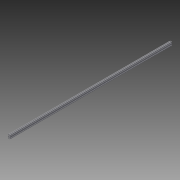
# Autodesk Inventor part: hfs5-2040
Saved by Autodesk Inventor 2013 (Build 170138000, 138)
## iProperties
Created: 2013-06-19
Part Number: hfs5-2040
Material: Generic
Document SubType Name: Modeling
Designer: Brett
Density: 1 g/cm^3
Author: Brett
Autodesk Inventor part; units mm, degrees
ref_plane "YZ Plane" through (0, 0, 0) normal (1, 0, 0) x (0, 1, 0)
ref_plane "XZ Plane" through (0, 0, 0) normal (0, 1, 0) x (-1, 0, 0)
ref_plane "XY Plane" through (0, 0, 0) normal (0, 0, 1) x (1, 0, 0)
sketch "Sketch1" plane through (0, 0, 0) normal (0, 0, 1) x (1, 0, 0)
  circle A0 centre (0, -10) radius 2.1
  circle A1 centre (0, 10) radius 2.1
  line L0 (-8, -6.7) -> (-8, -4)
  line L1 (-8, -4) -> (-7.0607, -4)
  line L2 (-7.0607, -4) -> (-4, -7.0607)
  line L3 (-4, -7.0607) -> (-4, -7.5)
  line L4 (-4, -7.5) -> (-3.751, -8.7811)
  line L5 (-3.751, -8.7811) -> (-3.933, -9.0964)
  arc A2 (-3.933, -9.0964) -> (-3.933, -9.5964) centre (-3.5, -9.3464) ccw
  line L6 (-3.933, -9.5964) -> (-3.7, -10)
  line L7 (-3.7, -10) -> (-3.933, -10.4036)
  arc A3 (-3.933, -10.4036) -> (-4, -10.6536) centre (-3.5, -10.6536) ccw
  line L8 (-4, -10.6536) -> (-4, -12.9393)
  line L9 (-4, -12.9393) -> (-7.0607, -16)
  line L10 (-7.0607, -16) -> (-8, -16)
  line L11 (-8, -16) -> (-8, -13.3)
  arc A4 (-8, -13.3) -> (-8.3, -13) centre (-8.3, -13.3) ccw
  line L12 (-8.3, -13) -> (-9.7, -13)
  arc A5 (-9.7, -13) -> (-10, -13.3) centre (-9.7, -13.3) ccw
  line L13 (-10, -13.3) -> (-10, -19)
  arc A6 (-10, -19) -> (-9, -20) centre (-9, -19) ccw
  line L14 (-9, -20) -> (-3.3, -20)
  arc A7 (-3.3, -20) -> (-3, -19.7) centre (-3.3, -19.7) ccw
  line L15 (-3, -19.7) -> (-3, -18.3)
  arc A8 (-3, -18.3) -> (-3.3, -18) centre (-3.3, -18.3) ccw
  line L16 (-3.3, -18) -> (-6, -18)
  line L17 (-6, -18) -> (-6, -17.0607)
  line L18 (-6, -17.0607) -> (-2.9393, -14)
  line L19 (-2.9393, -14) -> (-2.5, -14)
  line L20 (-2.5, -14) -> (-1.2189, -13.751)
  line L21 (-1.2189, -13.751) -> (-0.9036, -13.933)
  arc A9 (-0.9036, -13.933) -> (-0.4036, -13.933) centre (-0.6536, -13.5) ccw
  line L22 (-0.4036, -13.933) -> (0, -13.7)
  line L23 (0, -13.7) -> (0.4036, -13.933)
  arc A10 (0.4036, -13.933) -> (0.9036, -13.933) centre (0.6536, -13.5) ccw
  line L24 (0.9036, -13.933) -> (1.2189, -13.751)
  line L25 (1.2189, -13.751) -> (2.5, -14)
  line L26 (2.5, -14) -> (2.9393, -14)
  line L27 (2.9393, -14) -> (6, -17.0607)
  line L28 (6, -17.0607) -> (6, -18)
  line L29 (6, -18) -> (3.3, -18)
  arc A11 (3.3, -18) -> (3, -18.3) centre (3.3, -18.3) ccw
  line L30 (3, -18.3) -> (3, -19.7)
  arc A12 (3, -19.7) -> (3.3, -20) centre (3.3, -19.7) ccw
  line L31 (3.3, -20) -> (9, -20)
  arc A13 (9, -20) -> (10, -19) centre (9, -19) ccw
  line L32 (10, -19) -> (10, -13.3)
  arc A14 (10, -13.3) -> (9.7, -13) centre (9.7, -13.3) ccw
  line L33 (9.7, -13) -> (8.3, -13)
  arc A15 (8.3, -13) -> (8, -13.3) centre (8.3, -13.3) ccw
  line L34 (8, -13.3) -> (8, -16)
  line L35 (8, -16) -> (7.0607, -16)
  line L36 (7.0607, -16) -> (4, -12.9393)
  line L37 (4, -12.9393) -> (4, -10.6536)
  arc A16 (4, -10.6536) -> (3.933, -10.4036) centre (3.5, -10.6536) ccw
  line L38 (3.933, -10.4036) -> (3.7, -10)
  line L39 (3.7, -10) -> (3.933, -9.5964)
  arc A17 (3.933, -9.5964) -> (3.933, -9.0964) centre (3.5, -9.3464) ccw
  line L40 (3.933, -9.0964) -> (3.751, -8.7811)
  line L41 (3.751, -8.7811) -> (4, -7.5)
  line L42 (4, -7.5) -> (4, -7.0607)
  line L43 (4, -7.0607) -> (7.0607, -4)
  line L44 (7.0607, -4) -> (8, -4)
  line L45 (8, -4) -> (8, -6.7)
  arc A18 (8, -6.7) -> (8.3, -7) centre (8.3, -6.7) ccw
  line L46 (8.3, -7) -> (9.7, -7)
  arc A19 (9.7, -7) -> (10, -6.7) centre (9.7, -6.7) ccw
  line L47 (10, -6.7) -> (10, 6.7)
  arc A20 (10, 6.7) -> (9.7, 7) centre (9.7, 6.7) ccw
  line L48 (9.7, 7) -> (8.3, 7)
  arc A21 (8.3, 7) -> (8, 6.7) centre (8.3, 6.7) ccw
  line L49 (8, 6.7) -> (8, 4)
  line L50 (8, 4) -> (7.0607, 4)
  line L51 (7.0607, 4) -> (4, 7.0607)
  line L52 (4, 7.0607) -> (4, 9.3464)
  arc A22 (4, 9.3464) -> (3.933, 9.5964) centre (3.5, 9.3464) ccw
  line L53 (3.933, 9.5964) -> (3.7, 10)
  line L54 (3.7, 10) -> (3.933, 10.4036)
  arc A23 (3.933, 10.4036) -> (3.933, 10.9036) centre (3.5, 10.6536) ccw
  line L55 (3.933, 10.9036) -> (3.751, 11.2189)
  line L56 (3.751, 11.2189) -> (4, 12.5)
  line L57 (4, 12.5) -> (4, 12.9393)
  line L58 (4, 12.9393) -> (7.0607, 16)
  line L59 (7.0607, 16) -> (8, 16)
  line L60 (8, 16) -> (8, 13.3)
  arc A24 (8, 13.3) -> (8.3, 13) centre (8.3, 13.3) ccw
  line L61 (8.3, 13) -> (9.7, 13)
  arc A25 (9.7, 13) -> (10, 13.3) centre (9.7, 13.3) ccw
  line L62 (10, 13.3) -> (10, 19)
  arc A26 (10, 19) -> (9, 20) centre (9, 19) ccw
  line L63 (9, 20) -> (3.3, 20)
  arc A27 (3.3, 20) -> (3, 19.7) centre (3.3, 19.7) ccw
  line L64 (3, 19.7) -> (3, 18.3)
  arc A28 (3, 18.3) -> (3.3, 18) centre (3.3, 18.3) ccw
  line L65 (3.3, 18) -> (6, 18)
  line L66 (6, 18) -> (6, 17.0607)
  line L67 (6, 17.0607) -> (2.9393, 14)
  line L68 (2.9393, 14) -> (0.6536, 14)
  arc A29 (0.6536, 14) -> (0.4036, 13.933) centre (0.6536, 13.5) ccw
  line L69 (0.4036, 13.933) -> (0, 13.7)
  line L70 (0, 13.7) -> (-0.6536, 14)
  line L71 (-0.6536, 14) -> (-2.9393, 14)
  line L72 (-2.9393, 14) -> (-6, 17.0607)
  line L73 (-6, 17.0607) -> (-6, 18)
  line L74 (-6, 18) -> (-3.3, 18)
  arc A30 (-3.3, 18) -> (-3, 18.3) centre (-3.3, 18.3) ccw
  line L75 (-3, 18.3) -> (-3, 19.7)
  arc A31 (-3, 19.7) -> (-3.3, 20) centre (-3.3, 19.7) ccw
  line L76 (-3.3, 20) -> (-9, 20)
  arc A32 (-9, 20) -> (-10, 19) centre (-9, 19) ccw
  line L77 (-10, 19) -> (-10, 13.3)
  arc A33 (-10, 13.3) -> (-9.7, 13) centre (-9.7, 13.3) ccw
  line L78 (-9.7, 13) -> (-8.3, 13)
  arc A34 (-8.3, 13) -> (-8, 13.3) centre (-8.3, 13.3) ccw
  line L79 (-8, 13.3) -> (-8, 16)
  line L80 (-8, 16) -> (-7.0607, 16)
  line L81 (-7.0607, 16) -> (-4, 12.9393)
  line L82 (-4, 12.9393) -> (-4, 12.5)
  line L83 (-4, 12.5) -> (-3.751, 11.2189)
  line L84 (-3.751, 11.2189) -> (-3.933, 10.9036)
  arc A35 (-3.933, 10.9036) -> (-3.933, 10.4036) centre (-3.5, 10.6536) ccw
  line L85 (-3.933, 10.4036) -> (-3.7, 10)
  line L86 (-3.7, 10) -> (-3.933, 9.5964)
  arc A36 (-3.933, 9.5964) -> (-4, 9.3464) centre (-3.5, 9.3464) ccw
  line L87 (-4, 9.3464) -> (-4, 7.0607)
  line L88 (-4, 7.0607) -> (-7.0607, 4)
  line L89 (-7.0607, 4) -> (-8, 4)
  line L90 (-8, 4) -> (-8, 6.7)
  arc A37 (-8, 6.7) -> (-8.3, 7) centre (-8.3, 6.7) ccw
  line L91 (-8.3, 7) -> (-9.7, 7)
  arc A38 (-9.7, 7) -> (-10, 6.7) centre (-9.7, 6.7) ccw
  line L92 (-10, 6.7) -> (-10, -6.7)
  arc A39 (-10, -6.7) -> (-9.7, -7) centre (-9.7, -6.7) ccw
  line L93 (-9.7, -7) -> (-8.3, -7)
  arc A40 (-8.3, -7) -> (-8, -6.7) centre (-8.3, -6.7) ccw
  line L94 (2.9393, 6) -> (6.8515, 2.0879)
  arc A41 (6.8515, 2.0879) -> (7.0636, 2) centre (7.0636, 2.3) ccw
  line L95 (7.0636, 2) -> (7.7, 2)
  arc A42 (8, 1.7) -> (7.7, 2) centre (7.7, 1.7) ccw
  line L96 (8, 1.7) -> (8, -1.7)
  arc A43 (7.7, -2) -> (8, -1.7) centre (7.7, -1.7) ccw
  line L97 (7.7, -2) -> (7.0636, -2)
  arc A44 (7.0636, -2) -> (6.8515, -2.0879) centre (7.0636, -2.3) ccw
  line L98 (6.8515, -2.0879) -> (2.9393, -6)
  line L99 (2.9393, -6) -> (0, -6)
  line L100 (0, -6) -> (-2.9393, -6)
  line L101 (-2.9393, -6) -> (-6.8515, -2.0879)
  arc A45 (-6.8515, -2.0879) -> (-7.0636, -2) centre (-7.0636, -2.3) ccw
  line L102 (-7.0636, -2) -> (-7.7, -2)
  arc A46 (-8, -1.7) -> (-7.7, -2) centre (-7.7, -1.7) ccw
  line L103 (-8, -1.7) -> (-8, 1.7)
  arc A47 (-7.7, 2) -> (-8, 1.7) centre (-7.7, 1.7) ccw
  line L104 (-7.7, 2) -> (-7.0636, 2)
  arc A48 (-7.0636, 2) -> (-6.8515, 2.0879) centre (-7.0636, 2.3) ccw
  line L105 (-6.8515, 2.0879) -> (-2.9393, 6)
  line L106 (-2.9393, 6) -> (0, 6)
  line L107 (0, 6) -> (2.9393, 6)
  constraints: 216 end point, 167 tangent, 94 point on circle, 49 centre point, 44 equal radius, 44 parallel, 30 perpendicular, 5 collinear
extrude "Extrusion1" add sketch "Sketch1" along normal blind 1800
body "Solid1"
